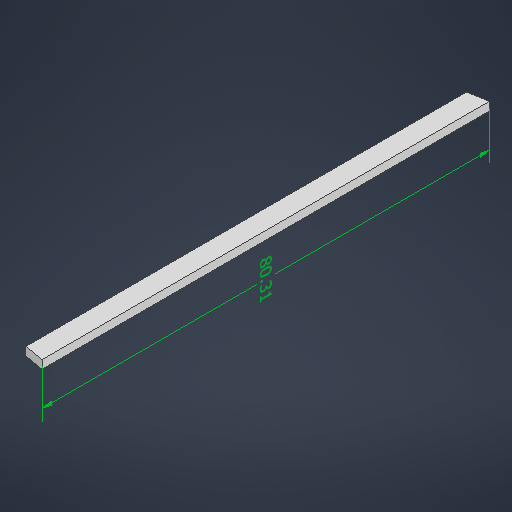
# Autodesk Inventor part: S_2x4x80.31
Saved by Autodesk Inventor 2027.1 (Build 311270010, 270A)
## iProperties
Created: 2026-09-04
Part Number: S_2x4x80.31
Material: Generic
Document SubType Name: Modeling
Designer: jorda
Density: 1 g/cm^3
Appearance: Default
Author: jorda
Autodesk Inventor part; units mm, degrees
ref_plane "YZ Plane" through (0, 0, 0) normal (1, 0, 0) x (0, 1, 0)
ref_plane "XZ Plane" through (0, 0, 0) normal (0, 1, 0) x (-1, 0, 0)
ref_plane "XY Plane" through (0, 0, 0) normal (0, 0, 1) x (1, 0, 0)
sketch "Sketch1" plane through (0, 0, 0) normal (0, 1, 0) x (-1, 0, 0)
  line L0 (1219.2, -214.9779) -> (1219.2, -2223.4221)
  line L1 (1130.3, -1062.1997) -> (1130.3, -2239.0976)
  line L2 (1130.3, -2239.0976) -> (1130.3, -199.3024)
  line L3 (1130.3, -199.3024) -> (1219.2, -214.9779)
  line L4 (1219.2, -214.9779) -> (1219.2, -2223.4221)
  line L5 (1130.3, -2239.0976) -> (1219.2, -2223.4221)
  point P0 (0, 0)
  constraints: 12 end point
extrude "Extrusion1" add sketch "Sketch1" along normal blind 38.1
body "Solid1"
